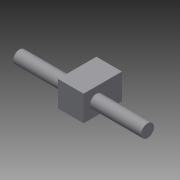
# Autodesk Inventor part: Cart Handle Pivot
Saved by Autodesk Inventor 2014 SP1 (Build 180222100, 222)
## iProperties
Created: 2014-02-04
Part Number: Cart Handle Pivot
Material: Generic
Document SubType Name: Modeling
Designer: Nitesh
Density: 1 g/cm^3
Appearance: Default
Mass: 37.451 g
Surface Area: 92.1494 cm^2
Volume: 37.451 cm^3
Author: Nitesh
Autodesk Inventor part; units mm, degrees
ref_plane "YZ Plane" through (0, 0, 0) normal (1, 0, 0) x (0, 1, 0)
ref_plane "XZ Plane" through (0, 0, 0) normal (0, 1, 0) x (-1, 0, 0)
ref_plane "XY Plane" through (0, 0, 0) normal (0, 0, 1) x (1, 0, 0)
sketch "Sketch1" plane through (0, 0, 0) normal (1, 0, 0) x (0, 1, 0)
  line L0 (0, 0) -> (25.4, 0)
  line L1 (25.4, 0) -> (25.4, 38.1)
  line L2 (25.4, 38.1) -> (0, 38.1)
  line L3 (0, 38.1) -> (0, 0)
  dimension "d0" = 38.1
  dimension "d1" = 25.4
  constraints: 8 end point, 2 parallel, 1 horizontal, 1 perpendicular
  measures "d0" distance of L2.end L0.start
  measures "d1" distance of L0.start L0.end
extrude "Extrusion1" add sketch "Sketch1" along normal blind 25.4
sketch "Sketch2" plane through (0, 0, 0) normal (-1, 0, 0) x (0, 0, 1)
  line L0 (0, 0) -> (0, 25.4) projected
  line L1 (0, 25.4) -> (38.1, 25.4) projected
  circle A0 centre (25.4, 12.7) radius 6.35
  dimension "d7" = 12.7
  dimension "d8" = 12.7
  dimension "d9" = 25.4
  constraints: 1 centre point
  measures "d7" diameter of A0
  measures "d8" distance from line of L1 A0.centre
  measures "d9" distance from line of L0 A0.centre
extrude "Extrusion2" add sketch "Sketch2" along normal blind 50.8 and the other way blind 76.2
body "Solid1"
